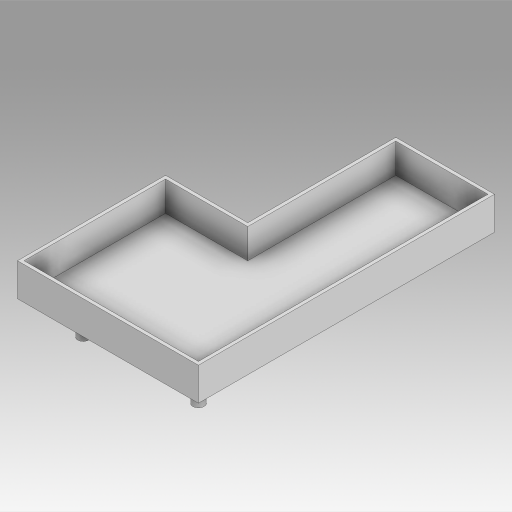
# Autodesk Inventor part: skrzynka_na_elektronike
Saved by Autodesk Inventor 2024.3 (Build 283343000, 343)
## iProperties
Created: 2025-10-17
Part Number: skrzynka_na_elektronike
Material: Ogólny
Document SubType Name: Modeling
Designer: User
Density: 1 g/cm^3
Appearance: Domyślna
Author: User
Autodesk Inventor part; units mm, degrees
ref_plane "YZ Plane" through (0, 0, 0) normal (1, 0, 0) x (0, 1, 0)
ref_plane "XZ Plane" through (0, 0, 0) normal (0, 1, 0) x (-1, 0, 0)
ref_plane "XY Plane" through (0, 0, 0) normal (0, 0, 1) x (1, 0, 0)
sketch "Szkic1" plane through (0, 0, 0) normal (0, 1, 0) x (-1, 0, 0)
  line L0 (0, 0) -> (110, 0)
  line L1 (110, 0) -> (110, -90)
  line L2 (110, -90) -> (0, -90)
  line L3 (0, -90) -> (0, 0)
  line L4 (0, -90) -> (60, -90)
  line L5 (60, -90) -> (60, -180)
  line L6 (60, -180) -> (0, -180)
  line L7 (0, -180) -> (0, -90)
  line L8 (2, -2) -> (108, -2)
  line L9 (108, -2) -> (108, -88)
  line L10 (108, -88) -> (2, -88)
  line L11 (2, -88) -> (2, -2)
  line L12 (2, -2) -> (108, -88) construction
  line L13 (108, -2) -> (2, -88) construction
  line L14 (2, -92) -> (58, -92)
  line L15 (58, -92) -> (58, -178)
  line L16 (58, -178) -> (2, -178)
  line L17 (2, -178) -> (2, -92)
  line L18 (2, -92) -> (58, -178) construction
  line L19 (58, -92) -> (2, -178) construction
  line L20 (55, -88) -> (2, -88)
  line L21 (2, -88) -> (2, -92)
  line L22 (2, -92) -> (55, -92)
  line L23 (55, -92) -> (55, -88)
  line L24 (58, -92) -> (2, -92)
  line L25 (2, -92) -> (2, -88)
  line L26 (2, -88) -> (58, -88)
  line L27 (58, -88) -> (58, -92)
  line L28 (0, 0) -> (10, 0)
  line L29 (10, 0) -> (10, -10)
  circle A0 centre (10, -10) radius 1.75
  circle A1 centre (10, -10) radius 3.5
  circle A2 centre (20, -10) radius 3.5
  circle A3 centre (20, -10) radius 1.75
  circle A4 centre (30, -10) radius 3.5
  circle A5 centre (30, -10) radius 1.75
  circle A6 centre (40, -10) radius 3.5
  circle A7 centre (40, -10) radius 1.75
  circle A8 centre (50, -10) radius 3.5
  circle A9 centre (50, -10) radius 1.75
  circle A10 centre (60, -10) radius 3.5
  circle A11 centre (60, -10) radius 1.75
  circle A12 centre (70, -10) radius 3.5
  circle A13 centre (70, -10) radius 1.75
  circle A14 centre (80, -10) radius 3.5
  circle A15 centre (80, -10) radius 1.75
  circle A16 centre (90, -10) radius 3.5
  circle A17 centre (90, -10) radius 1.75
  circle A18 centre (100, -10) radius 3.5
  circle A19 centre (100, -10) radius 1.75
  circle A20 centre (10, -20) radius 3.5
  circle A21 centre (10, -20) radius 1.75
  circle A22 centre (20, -20) radius 3.5
  circle A23 centre (20, -20) radius 1.75
  circle A24 centre (30, -20) radius 3.5
  circle A25 centre (30, -20) radius 1.75
  circle A26 centre (40, -20) radius 3.5
  circle A27 centre (40, -20) radius 1.75
  circle A28 centre (50, -20) radius 3.5
  circle A29 centre (50, -20) radius 1.75
  circle A30 centre (60, -20) radius 3.5
  circle A31 centre (60, -20) radius 1.75
  circle A32 centre (70, -20) radius 3.5
  circle A33 centre (70, -20) radius 1.75
  circle A34 centre (80, -20) radius 3.5
  circle A35 centre (80, -20) radius 1.75
  circle A36 centre (90, -20) radius 3.5
  circle A37 centre (90, -20) radius 1.75
  circle A38 centre (100, -20) radius 3.5
  circle A39 centre (100, -20) radius 1.75
  circle A40 centre (10, -30) radius 3.5
  circle A41 centre (10, -30) radius 1.75
  circle A42 centre (20, -30) radius 3.5
  circle A43 centre (20, -30) radius 1.75
  circle A44 centre (30, -30) radius 3.5
  circle A45 centre (30, -30) radius 1.75
  circle A46 centre (40, -30) radius 3.5
  circle A47 centre (40, -30) radius 1.75
  circle A48 centre (50, -30) radius 3.5
  circle A49 centre (50, -30) radius 1.75
  circle A50 centre (60, -30) radius 3.5
  circle A51 centre (60, -30) radius 1.75
  circle A52 centre (70, -30) radius 3.5
  circle A53 centre (70, -30) radius 1.75
  circle A54 centre (80, -30) radius 3.5
  circle A55 centre (80, -30) radius 1.75
  circle A56 centre (90, -30) radius 3.5
  circle A57 centre (90, -30) radius 1.75
  circle A58 centre (100, -30) radius 3.5
  circle A59 centre (100, -30) radius 1.75
  circle A60 centre (10, -40) radius 3.5
  circle A61 centre (10, -40) radius 1.75
  circle A62 centre (20, -40) radius 3.5
  circle A63 centre (20, -40) radius 1.75
  circle A64 centre (30, -40) radius 3.5
  circle A65 centre (30, -40) radius 1.75
  circle A66 centre (40, -40) radius 3.5
  circle A67 centre (40, -40) radius 1.75
  circle A68 centre (50, -40) radius 3.5
  circle A69 centre (50, -40) radius 1.75
  circle A70 centre (60, -40) radius 3.5
  circle A71 centre (60, -40) radius 1.75
  circle A72 centre (70, -40) radius 3.5
  circle A73 centre (70, -40) radius 1.75
  circle A74 centre (80, -40) radius 3.5
  circle A75 centre (80, -40) radius 1.75
  circle A76 centre (90, -40) radius 3.5
  circle A77 centre (90, -40) radius 1.75
  circle A78 centre (100, -40) radius 3.5
  circle A79 centre (100, -40) radius 1.75
  circle A80 centre (10, -50) radius 3.5
  circle A81 centre (10, -50) radius 1.75
  circle A82 centre (20, -50) radius 3.5
  circle A83 centre (20, -50) radius 1.75
  circle A84 centre (30, -50) radius 3.5
  circle A85 centre (30, -50) radius 1.75
  circle A86 centre (40, -50) radius 3.5
  circle A87 centre (40, -50) radius 1.75
  circle A88 centre (50, -50) radius 3.5
  circle A89 centre (50, -50) radius 1.75
  circle A90 centre (60, -50) radius 3.5
  circle A91 centre (60, -50) radius 1.75
  circle A92 centre (70, -50) radius 3.5
  circle A93 centre (70, -50) radius 1.75
  circle A94 centre (80, -50) radius 3.5
  circle A95 centre (80, -50) radius 1.75
  circle A96 centre (90, -50) radius 3.5
  circle A97 centre (90, -50) radius 1.75
  circle A98 centre (100, -50) radius 3.5
  circle A99 centre (100, -50) radius 1.75
  circle A100 centre (10, -60) radius 3.5
  circle A101 centre (10, -60) radius 1.75
  circle A102 centre (20, -60) radius 3.5
  circle A103 centre (20, -60) radius 1.75
  circle A104 centre (30, -60) radius 3.5
  circle A105 centre (30, -60) radius 1.75
  circle A106 centre (40, -60) radius 3.5
  circle A107 centre (40, -60) radius 1.75
  circle A108 centre (50, -60) radius 3.5
  circle A109 centre (50, -60) radius 1.75
  circle A110 centre (60, -60) radius 3.5
  circle A111 centre (60, -60) radius 1.75
  circle A112 centre (70, -60) radius 3.5
  circle A113 centre (70, -60) radius 1.75
  circle A114 centre (80, -60) radius 3.5
  circle A115 centre (80, -60) radius 1.75
  circle A116 centre (90, -60) radius 3.5
  circle A117 centre (90, -60) radius 1.75
  circle A118 centre (100, -60) radius 3.5
  circle A119 centre (100, -60) radius 1.75
  circle A120 centre (10, -70) radius 3.5
  circle A121 centre (10, -70) radius 1.75
  circle A122 centre (20, -70) radius 3.5
  circle A123 centre (20, -70) radius 1.75
  circle A124 centre (30, -70) radius 3.5
  circle A125 centre (30, -70) radius 1.75
  circle A126 centre (40, -70) radius 3.5
  circle A127 centre (40, -70) radius 1.75
  circle A128 centre (50, -70) radius 3.5
  circle A129 centre (50, -70) radius 1.75
  circle A130 centre (60, -70) radius 3.5
  circle A131 centre (60, -70) radius 1.75
  circle A132 centre (70, -70) radius 3.5
  circle A133 centre (70, -70) radius 1.75
  circle A134 centre (80, -70) radius 3.5
  circle A135 centre (80, -70) radius 1.75
  circle A136 centre (90, -70) radius 3.5
  circle A137 centre (90, -70) radius 1.75
  circle A138 centre (100, -70) radius 3.5
  circle A139 centre (100, -70) radius 1.75
  circle A140 centre (10, -80) radius 3.5
  circle A141 centre (10, -80) radius 1.75
  circle A142 centre (20, -80) radius 3.5
  circle A143 centre (20, -80) radius 1.75
  circle A144 centre (30, -80) radius 3.5
  circle A145 centre (30, -80) radius 1.75
  circle A146 centre (40, -80) radius 3.5
  circle A147 centre (40, -80) radius 1.75
  circle A148 centre (50, -80) radius 3.5
  circle A149 centre (50, -80) radius 1.75
  circle A150 centre (60, -80) radius 3.5
  circle A151 centre (60, -80) radius 1.75
  circle A152 centre (70, -80) radius 3.5
  circle A153 centre (70, -80) radius 1.75
  circle A154 centre (80, -80) radius 3.5
  circle A155 centre (80, -80) radius 1.75
  circle A156 centre (90, -80) radius 3.5
  circle A157 centre (90, -80) radius 1.75
  circle A158 centre (100, -80) radius 3.5
  circle A159 centre (100, -80) radius 1.75
  circle A160 centre (10, -90) radius 3.5
  circle A161 centre (10, -90) radius 1.75
  circle A162 centre (20, -90) radius 3.5
  circle A163 centre (20, -90) radius 1.75
  circle A164 centre (30, -90) radius 3.5
  circle A165 centre (30, -90) radius 1.75
  circle A166 centre (40, -90) radius 3.5
  circle A167 centre (40, -90) radius 1.75
  circle A168 centre (50, -90) radius 3.5
  circle A169 centre (50, -90) radius 1.75
  circle A170 centre (60, -90) radius 3.5
  circle A171 centre (60, -90) radius 1.75
  circle A172 centre (70, -90) radius 3.5
  circle A173 centre (70, -90) radius 1.75
  circle A174 centre (80, -90) radius 3.5
  circle A175 centre (80, -90) radius 1.75
  circle A176 centre (90, -90) radius 3.5
  circle A177 centre (90, -90) radius 1.75
  circle A178 centre (100, -90) radius 3.5
  circle A179 centre (100, -90) radius 1.75
  circle A180 centre (10, -100) radius 3.5
  circle A181 centre (10, -100) radius 1.75
  circle A182 centre (20, -100) radius 3.5
  circle A183 centre (20, -100) radius 1.75
  circle A184 centre (30, -100) radius 3.5
  circle A185 centre (30, -100) radius 1.75
  circle A186 centre (40, -100) radius 3.5
  circle A187 centre (40, -100) radius 1.75
  circle A188 centre (50, -100) radius 3.5
  circle A189 centre (50, -100) radius 1.75
  circle A190 centre (60, -100) radius 3.5
  circle A191 centre (60, -100) radius 1.75
  circle A192 centre (70, -100) radius 3.5
  circle A193 centre (70, -100) radius 1.75
  circle A194 centre (80, -100) radius 3.5
  circle A195 centre (80, -100) radius 1.75
  circle A196 centre (90, -100) radius 3.5
  circle A197 centre (90, -100) radius 1.75
  circle A198 centre (100, -100) radius 3.5
  circle A199 centre (100, -100) radius 1.75
  circle A200 centre (10, -110) radius 3.5
  circle A201 centre (10, -110) radius 1.75
  circle A202 centre (20, -110) radius 3.5
  circle A203 centre (20, -110) radius 1.75
  circle A204 centre (30, -110) radius 3.5
  circle A205 centre (30, -110) radius 1.75
  circle A206 centre (40, -110) radius 3.5
  circle A207 centre (40, -110) radius 1.75
  circle A208 centre (50, -110) radius 3.5
  circle A209 centre (50, -110) radius 1.75
  circle A210 centre (60, -110) radius 3.5
  circle A211 centre (60, -110) radius 1.75
  circle A212 centre (70, -110) radius 3.5
  circle A213 centre (70, -110) radius 1.75
  circle A214 centre (80, -110) radius 3.5
  circle A215 centre (80, -110) radius 1.75
  circle A216 centre (90, -110) radius 3.5
  circle A217 centre (90, -110) radius 1.75
  circle A218 centre (100, -110) radius 3.5
  circle A219 centre (100, -110) radius 1.75
  circle A220 centre (10, -120) radius 3.5
  circle A221 centre (10, -120) radius 1.75
  circle A222 centre (20, -120) radius 3.5
  circle A223 centre (20, -120) radius 1.75
  circle A224 centre (30, -120) radius 3.5
  circle A225 centre (30, -120) radius 1.75
  circle A226 centre (40, -120) radius 3.5
  circle A227 centre (40, -120) radius 1.75
  circle A228 centre (50, -120) radius 3.5
  circle A229 centre (50, -120) radius 1.75
  circle A230 centre (60, -120) radius 3.5
  circle A231 centre (60, -120) radius 1.75
  circle A232 centre (70, -120) radius 3.5
  circle A233 centre (70, -120) radius 1.75
  circle A234 centre (80, -120) radius 3.5
  circle A235 centre (80, -120) radius 1.75
  circle A236 centre (90, -120) radius 3.5
  circle A237 centre (90, -120) radius 1.75
  circle A238 centre (100, -120) radius 3.5
  circle A239 centre (100, -120) radius 1.75
  circle A240 centre (10, -130) radius 3.5
  circle A241 centre (10, -130) radius 1.75
  circle A242 centre (20, -130) radius 3.5
  circle A243 centre (20, -130) radius 1.75
  circle A244 centre (30, -130) radius 3.5
  circle A245 centre (30, -130) radius 1.75
  circle A246 centre (40, -130) radius 3.5
  circle A247 centre (40, -130) radius 1.75
  circle A248 centre (50, -130) radius 3.5
  circle A249 centre (50, -130) radius 1.75
  circle A250 centre (60, -130) radius 3.5
  circle A251 centre (60, -130) radius 1.75
  circle A252 centre (70, -130) radius 3.5
  circle A253 centre (70, -130) radius 1.75
  circle A254 centre (80, -130) radius 3.5
  circle A255 centre (80, -130) radius 1.75
  circle A256 centre (90, -130) radius 3.5
  circle A257 centre (90, -130) radius 1.75
  circle A258 centre (100, -130) radius 3.5
  circle A259 centre (100, -130) radius 1.75
  circle A260 centre (10, -140) radius 3.5
  circle A261 centre (10, -140) radius 1.75
  circle A262 centre (20, -140) radius 3.5
  circle A263 centre (20, -140) radius 1.75
  circle A264 centre (30, -140) radius 3.5
  circle A265 centre (30, -140) radius 1.75
  circle A266 centre (40, -140) radius 3.5
  circle A267 centre (40, -140) radius 1.75
  circle A268 centre (50, -140) radius 3.5
  circle A269 centre (50, -140) radius 1.75
  circle A270 centre (60, -140) radius 3.5
  circle A271 centre (60, -140) radius 1.75
  circle A272 centre (70, -140) radius 3.5
  circle A273 centre (70, -140) radius 1.75
  circle A274 centre (80, -140) radius 3.5
  circle A275 centre (80, -140) radius 1.75
  circle A276 centre (90, -140) radius 3.5
  circle A277 centre (90, -140) radius 1.75
  circle A278 centre (100, -140) radius 3.5
  circle A279 centre (100, -140) radius 1.75
  circle A280 centre (10, -150) radius 3.5
  circle A281 centre (10, -150) radius 1.75
  circle A282 centre (20, -150) radius 3.5
  circle A283 centre (20, -150) radius 1.75
  circle A284 centre (30, -150) radius 3.5
  circle A285 centre (30, -150) radius 1.75
  circle A286 centre (40, -150) radius 3.5
  circle A287 centre (40, -150) radius 1.75
  circle A288 centre (50, -150) radius 3.5
  circle A289 centre (50, -150) radius 1.75
  circle A290 centre (60, -150) radius 3.5
  circle A291 centre (60, -150) radius 1.75
  circle A292 centre (70, -150) radius 3.5
  circle A293 centre (70, -150) radius 1.75
  circle A294 centre (80, -150) radius 3.5
  circle A295 centre (80, -150) radius 1.75
  circle A296 centre (90, -150) radius 3.5
  circle A297 centre (90, -150) radius 1.75
  circle A298 centre (100, -150) radius 3.5
  circle A299 centre (100, -150) radius 1.75
  point P0 (55, -45)
  point P1 (30, -135)
  point P2 (60, -90)
  dimension "d0" = 110
  dimension "d1" = 90
  dimension "d2" = 60
  dimension "d3" = 90
  dimension "d4" = 106
  dimension "d5" = 86
  dimension "d6" = 56
  dimension "d7" = 86
  dimension "d12" = 10
  dimension "d13" = 10
  dimension "d14" = 90
  dimension "d15" = 3.5
  dimension "d16" = 7
  dimension "d19" = 10
  dimension "d22" = 10
  dimension "d27" = 2
  dimension "d28" = 2
  dimension "d29" = 2
  dimension "d30" = 2
  constraints: 300 centre point, 151 coincident, 60 end point, 12 parallel, 7 horizontal, 7 perpendicular, 5 midpoint, 1 point on line, 1 vertical, 596 other
  measures "d0" distance of L1.end L2.end
  measures "d1" distance of L0.end L1.end
  measures "d2" distance of L5.end L6.end
  measures "d3" distance of L4.end L5.end
  measures "d4" distance of L9.end L10.end
  measures "d5" distance of L8.end L9.end
  measures "d6" distance of L15.end L16.end
  measures "d7" distance of L14.end L15.end
  measures "d12" distance of L0.start L28.end
  measures "d13" distance of L28.end L29.end
  measures "d14" angle of L28 L29
  measures "d15" diameter of A0
  measures "d16" diameter of A1
  measures "d19" distance of A1.centre A2.centre
  measures "d22" distance of A1.centre A20.centre
  measures "d27" distance between parallel lines of L3 L11
  measures "d28" distance between parallel lines of L0 L8
  measures "d29" distance between parallel lines of L7 L17
  measures "d30" distance between parallel lines of L6 L16
extrude "Wyciągnięcie proste1" add sketch "Szkic1" along normal blind 2 contours L0 L29 L8 L11 L21 L2 L3 | L0 L1 L2 A178 L10 L9 L8 L29 | L2 L21 L17 L16 L15 A290 L5 L6 L7 | L8 L9 L10 A178 A176 A174 A172 A170 A168 A166 A164 A162 A160 L11 | A0 | A1 | L21 L10 A160 L2 | L2 A160 L14 L21 | A160 L10 L2 A161 | L2 A161 A160 L14 | L14 A160 A162 A164 A166 A168 A170 L15 A190 A210 A230 A250 A270 A290 L16 L17 | L2 A179 A178 L10 | A161 L2 | L2 A161 | A160 L10 | L14 A160 | A290 L15 L5 A291 | L2 A179 | L10 A178 | L2 A176 L10 A178 | L10 A162 L2 A160 | A160 L2 A162 L14 | A291 L5 | A290 L15 | L2 A177 A176 L10 | A162 L10 | L10 A162 L2 A163 | A162 L2 A163 L14 | L14 A162 | L15 A270 L5 A290 | L10 A176 | L2 A177 | L2 A174 L10 A176 | L10 A164 L2 A162 | A162 L2 A164 L14 | A270 L15 | L15 A270 L5 A271 | L2 A175 A174 L10 | A163 L2 | L2 A163 | A164 L10 | L10 A164 L2 A165 | A164 L2 A165 L14 | L14 A164 | L15 A250 L5 A270 | A271 L5 | L10 A174 | L2 A175 | L2 A172 L10 A174 | L10 A166 L2 A164 | A164 L2 A166 L14 | A250 L15 | L15 A250 L5 A251 | L2 A173 A172 L10 | A166 L10 | L10 A166 L2 A167 | A165 L2 | L2 A165 | A166 L2 A167 L14 | L14 A166 | L15 A230 L5 A250 | L10 A172 | L2 A173 | L2 A170 L10 A172 | L10 A168 L2 A166 | A166 L2 A168 L14 | A230 L15 | L15 A230 L5 A231 | A251 L5 | L2 A171 L27 L10 A170 | A168 L10 | L10 A168 L2 A169 | A167 L2 | L2 A167 | A168 L2 A169 L14 | L14 A168 | L15 A210 L5 A230 | L10 A170 | L2 A171 | A170 L15 L27 L2 A171 L5 | L5 A190 L15 A170 | L10 L23 L2 A168 | A168 L2 L23 L14 | A210 L15 | L15 A210 L5 A211 | A231 L5 | L27 L2 A170 L10 | A170 L2 L23 L10 | L5 A171 L2 | L5 A191 A190 L15 | A170 L14 L15 | A169 L2 | L2 A169 | L23 L2 A170 L14 | L15 A190 L5 A210 | L27 L14 A170 L2 | L5 A191 | L15 A190 | A211 L5 | A2 | A3 | A4 | A5 | A6 | A7 | A8 | A9 | A10 | A11 | A12 | A13 | A14 | A15 | A16 | A17 | A18 | A19 | A20 | A21 | A22 | A23 | A24 | A25 | A26 | A27 | A28 | A29 | A30 | A31 | A32 | A33 | A34 | A35 | A36 | A37 | A38 | A39 | A40 | A41 | A42 | A43 | A44 | A45 | A46 | A47 | A48 | A49 | A50 | A51 | A52 | A53 | A54 | A55 | A56 | A57 | A58 | A59 | A60 | A61 | A62 | A63 | A64 | A65 | A66 | A67 | A68 | A69 | A70 | A71 | A72 | A73 | A74 | A75 | A76 | A77 | A78 | A79 | A80 | A81 | A82 | A83 | A84 | A85 | A86 | A87 | A88 | A89 | A90 | A91 | A92 | A93 | A94 | A95 | A96 | A97 | A98 | A99 | A100 | A101 | A102 | A103 | A104 | A105 | A106 | A107 | A108 | A109 | A110 | A111 | A112 | A113 | A114 | A115 | A116 | A117 | A118 | A119 | A120 | A121 | A122 | A123 | A124 | A125 | A126 | A127 | A128 | A129 | A130 | A131 | A132 | A133 | A134 | A135 | A136 | A137 | A138 | A139 | A140 | A141 | A142 | A143 | A144 | A145 | A146 | A147 | A148 | A149 | A150 | A151 | A152 | A153 | A154 | A155 | A156 | A157 | A158 | A159 | A180 | A181 | A182 | A183 | A184 | A185 | A186 | A187 | A188 | A189 | A200 | A201 | A202 | A203 | A204 | A205 | A206 | A207 | A208 | A209 | A220 | A221 | A222 | A223 | A224 | A225 | A226 | A227 | A228 | A229 | A240 | A241 | A242 | A243 | A244 | A245 | A246 | A247 | A248 | A249 | A260 | A261 | A262 | A263 | A264 | A265 | A266 | A267 | A268 | A269 | A280 | A281 | A282 | A283 | A284 | A285 | A286 | A287 | A288 | A289 picked at (100.2069, -89.4546) picked at (59.4209, -150.0703) picked at (90.2069, -89.4546) picked at (59.4209, -140.0703) picked at (80.2069, -89.4546) picked at (70.2069, -89.4546) picked at (59.4209, -130.0703) picked at (59.5199, -120.3314) picked at (58.848, -90.1298) picked at (59.1092, -100.2815) picked at (59.5199, -110.3314)
extrude "Wyciągnięcie proste2" add sketch "Szkic1" along normal blind 20 contours L0 L29 L8 L11 L21 L2 L3 | L0 L1 L2 A178 L10 L9 L8 L29 | L2 L21 L17 L16 L15 A290 L5 L6 L7 | L2 A179 A178 L10 | A290 L15 L5 A291 | L2 A179 | L2 A176 L10 A178 | A291 L5 | L2 A177 A176 L10 | L15 A270 L5 A290 | L2 A177 | L2 A174 L10 A176 | L15 A270 L5 A271 | L2 A175 A174 L10 | L15 A250 L5 A270 | A271 L5 | L2 A175 | L2 A172 L10 A174 | L15 A250 L5 A251 | L2 A173 A172 L10 | L15 A230 L5 A250 | L2 A173 | L2 A170 L10 A172 | L15 A230 L5 A231 | A251 L5 | L2 A171 L27 L10 A170 | L15 A210 L5 A230 | L2 A171 | A170 L15 L27 L2 A171 L5 | L5 A190 L15 A170 | L15 A210 L5 A211 | A231 L5 | L5 A171 L2 | L5 A191 A190 L15 | L15 A190 L5 A210 | L5 A191 | A211 L5 picked at (100.2069, -89.4546) picked at (59.4209, -150.0703) picked at (90.2069, -89.4546) picked at (59.4209, -140.0703) picked at (80.2069, -89.4546) picked at (70.2069, -89.4546) picked at (59.4209, -130.0703) picked at (59.5199, -120.3314) picked at (58.848, -90.1298) picked at (59.1092, -100.2815) picked at (59.5199, -110.3314)
extrude "Wyciągnięcie proste3" add sketch "Szkic1" against normal blind 10 contours A1 | A14 | A284
